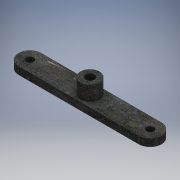
# Autodesk Inventor part: крышка
Saved by Autodesk Inventor 2018 (Build 220112000, 112)
## iProperties
Created: 2020-04-07
Part Number: крышка
Material: Сталь
Document SubType Name: ЛистМат
Designer: Nikita
Density: 7.85 g/cm^3
Appearance: Листовая
Sheet Metal Rule: По умолчанию_мм
Author: Nikita
Autodesk Inventor part; units mm, degrees
ref_plane "YZ Plane" through (0, 0, 0) normal (1, 0, 0) x (0, 1, 0)
ref_plane "XZ Plane" through (0, 0, 0) normal (0, 1, 0) x (-1, 0, 0)
ref_plane "XY Plane" through (0, 0, 0) normal (0, 0, 1) x (1, 0, 0)
sketch "Эскиз1" plane through (0, 0, 0) normal (0, 0, 1) x (1, 0, 0)
  line L0 (80, 0) -> (-80, 0) construction
  line L1 (80, 15) -> (-80, 15)
  line L2 (-80, -15) -> (80, -15)
  arc A0 (80, -15) -> (80, 15) centre (80, 0) ccw
  arc A1 (-80, 15) -> (-80, -15) centre (-80, 0) ccw
  circle A2 centre (0, 0) radius 12.5
  circle A3 centre (0, 0) radius 6
  circle A4 centre (-80, 0) radius 5
  circle A5 centre (80, 0) radius 5
  dimension "d0" = 80
  dimension "d1" = 30
  dimension "d4" = 25
  dimension "d5" = 12
  dimension "d6" = 10
  dimension "d7" = 10
  constraints: 8 end point, 6 centre point, 4 coincident, 4 point on circle, 4 tangent, 1 horizontal, 1 midpoint, 1 parallel
  measures "d0" distance of point (0, 0) L0.end
  measures "d1" diameter of A1
  measures "d4" diameter of A2
  measures "d5" diameter of A3
  measures "d6" diameter of A4
  measures "d7" diameter of A5
extrude "Выдавливание1" add sketch "Эскиз1" against normal blind 10 contours A0 L2 A1 L1 | A2 | A3 | A4 | A5
extrude "Выдавливание2" cut sketch "Эскиз1" against normal blind 10 contours A5
extrude "Выдавливание3" cut sketch "Эскиз1" against normal blind 10 contours A4
extrude "Выдавливание4" add sketch "Эскиз1" along normal blind 20 contours A2
extrude "Выдавливание5" cut sketch "Эскиз1" along normal mid plane 2850 contours A3
equation "\"Глубина_просечки\" = 0.5 * Толщина"
equation "\"Толщина\" = 10"
